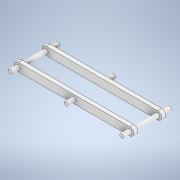
# Autodesk Inventor part: Joint 2
Saved by Autodesk Inventor 2021 (Build 250183000, 183)
## iProperties
Created: 2021-04-01
Part Number: Joint 2
Material: Generic
Document SubType Name: Modeling
Designer: Darek
Density: 1 g/cm^3
Appearance: Default
Mass: 17.1416 g
Surface Area: 108.347 cm^2
Volume: 17.1416 cm^3
Author: Darek
Autodesk Inventor part; units mm, degrees
ref_plane "YZ Plane" through (0, 0, 0) normal (1, 0, 0) x (0, 1, 0)
ref_plane "XZ Plane" through (0, 0, 0) normal (0, 1, 0) x (-1, 0, 0)
ref_plane "XY Plane" through (0, 0, 0) normal (0, 0, 1) x (1, 0, 0)
sketch "Sketch1" plane through (0, 0, 0) normal (0, 0, 1) x (1, 0, 0)
  line L0 (0, 0) -> (150, 0)
  line L1 (150, 0) -> (150, 10)
  line L2 (150, 10) -> (0, 10)
  line L3 (0, 10) -> (0, 0)
  dimension "d0" = 10
  dimension "d1" = 150
  constraints: 8 end point, 3 perpendicular, 1 horizontal
  measures "d0" distance between parallel lines of L0 L2
  measures "d1" distance between parallel lines of L3 L1
extrude "Extrusion1" add sketch "Sketch1" along normal blind 40
sketch "Sketch2" plane through (0, 10, 0) normal (0, 1, 0) x (1, 0, 0)
  line L0 (0, -35) -> (150, -35)
  line L1 (150, -35) -> (150, -5)
  line L2 (150, -5) -> (0, -5)
  line L3 (0, -5) -> (0, -35)
  line L4 (0, 0) -> (0, -40) projected
  line L5 (150, 0) -> (150, -40) projected
  line L6 (150, 0) -> (0, 0) projected
  line L7 (150, -40) -> (0, -40) projected
  dimension "d4" = 0
  dimension "d5" = 0
  dimension "d6" = 5
  dimension "d7" = 5
  constraints: 8 end point, 2 parallel, 1 horizontal, 1 perpendicular
  measures "d4" distance between parallel lines of L4 L3
  measures "d5" distance between parallel lines of L5 L1
  measures "d6" distance between parallel lines of L6 L2
  measures "d7" distance between parallel lines of L7 L0
extrude "Extrusion2" cut sketch "Sketch2" against normal blind 10 contours L3 L2 L1 L0
sketch "Sketch3" plane through (0, 10, 5) normal (0, 0, 1) x (1, 0, 0)
  point P0 (0, -10)
sketch "Sketch4" plane through (0, 0, 0) normal (0, 0, -1) x (-1, 0, 0)
  circle A0 centre (-5, 5) radius 2.5
  circle A1 centre (-145, 5) radius 2.5
  line L0 (-150, 0) -> (-150, 10) projected
  line L1 (0, 0) -> (-150, 0) projected
  line L2 (-150, 10) -> (0, 10) projected
  line L3 (0, 10) -> (0, 0) projected
  circle A2 centre (-75, 5) radius 2.5
  dimension "d10" = 5
  dimension "d11" = 5
  dimension "d12" = 5
  dimension "d13" = 5
  dimension "d14" = 5
  dimension "d15" = 5
  dimension "d21" = 70
  dimension "d22" = 5
  dimension "d23" = 5
  constraints: 3 centre point
  measures "d10" diameter of A1
  measures "d11" distance from line of L0 A1.centre
  measures "d12" distance from line of L1 A1.centre
  measures "d13" diameter of A0
  measures "d14" distance from line of L2 A0.centre
  measures "d15" distance from line of L3 A0.centre
  measures "d21" distance of A0.centre A2.centre
  measures "d22" diameter of A2
  measures "d23" distance from line of L1 A2.centre
extrude "Extrusion3" add sketch "Sketch4" along normal blind 10 and the other way blind 50 contours A0 | A1
fillet "Fillet1" radius 5 8 edges at (150, 10, 37.5) (150, 10, 2.5) (0, 10, 37.5) (0, 10, 2.5) (150, 0, 37.5) (150, 0, 2.5) (0, 0, 37.5) (0, 0, 2.5)
extrude "Extrusion4" add sketch "Sketch4" along normal blind 10 contours A2
sketch "Sketch5" plane through (0, 0, 40) normal (0, 0, 1) x (1, 0, 0)
  circle A0 centre (75, 5) radius 2.5
  circle A1 centre (5, 5) radius 2.5 projected
  line L0 (5, 0) -> (145, 0) projected
  point P0 (0, 0)
  dimension "d26" = 70
  dimension "d27" = 5
  dimension "d28" = 5
  constraints: 1 centre point
  measures "d26" distance of A1.centre A0.centre
  measures "d27" diameter of A0
  measures "d28" distance from line of L0 A0.centre
extrude "Extrusion5" add sketch "Sketch5" along normal blind 10 contours A0
body "Solid1"
